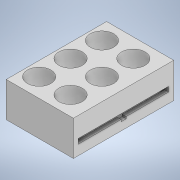
# Autodesk Inventor part: StirredVialHolder
Saved by Autodesk Inventor 2020 (Build 240168000, 168)
## iProperties
Created: 2021-07-14
Part Number: StirredVialHolder
Material: Generic
Document SubType Name: Modeling
Designer: pab2
Density: 1 g/cm^3
Appearance: Default
Author: pab2
Autodesk Inventor part; units mm, degrees
ref_plane "YZ Plane" through (0, 0, 0) normal (1, 0, 0) x (0, 1, 0)
ref_plane "XZ Plane" through (0, 0, 0) normal (0, 1, 0) x (-1, 0, 0)
ref_plane "XY Plane" through (0, 0, 0) normal (0, 0, 1) x (1, 0, 0)
sketch "Sketch1" plane through (0, 0, 0) normal (0, 1, 0) x (-1, 0, 0)
  line L0 (0, 0) -> (85.48, 0)
  line L1 (85.48, 0) -> (85.48, -127.76)
  line L2 (85.48, -127.76) -> (0, -127.76)
  line L3 (0, -127.76) -> (0, 0)
  line L4 (0, 0) -> (7.0711, -7.0711)
  line L5 (0, 0) -> (10, 0) construction
  circle A0 centre (7.0711, -7.0711) radius 4.7625
  dimension "d0" = 85.48
  dimension "d1" = 127.76
  dimension "offsetDiag" = 10
  dimension "d3" = 45
  dimension "d4" = 9.525
  constraints: 12 end point, 2 horizontal, 2 parallel, 1 centre point, 1 coincident, 1 equal length, 1 perpendicular
  measures "d0" distance of L1.end L2.end
  measures "d1" distance of L0.end L1.end
  measures "offsetDiag" distance of L0.start L4.end
  measures "d3" angle of L4 L5
  measures "d4" diameter of A0
extrude "Extrusion1" add sketch "Sketch1" along normal blind 12.7 contours L0 L1 L2 L3 | A0
sketch "Sketch3" plane through (0, 12.7, 0) normal (0, 1, 0) x (1, 0, 0)
  line L0 (0, 0) -> (0, 127.76) projected
  line L1 (0, 63.88) -> (-72.5, 63.88)
  line L2 (-140, 121.63) -> (-5, 121.63)
  line L3 (-5, 121.63) -> (-5, 6.13)
  line L4 (-5, 6.13) -> (-140, 6.13)
  line L5 (-140, 6.13) -> (-140, 121.63)
  line L6 (-140, 121.63) -> (-5, 6.13) construction
  line L7 (-5, 121.63) -> (-140, 6.13) construction
  dimension "d23" = 72.5
  dimension "d24" = 135
  dimension "d25" = 115.5
  constraints: 14 end point, 3 midpoint, 2 horizontal, 2 parallel, 1 perpendicular
  measures "d23" distance of L1.start L1.end
  measures "d24" distance of L3.end L4.end
  measures "d25" distance of L2.end L3.end
extrude "Extrusion2" cut sketch "Sketch3" against normal blind 2.54
sketch "Sketch4" plane through (0, 12.7, 0) normal (0, 1, 0) x (1, 0, 0)
  line L0 (-5, 121.63) -> (-5, 6.13) projected
  line L1 (5, 67.055) -> (-5, 67.055)
  line L2 (-5, 67.055) -> (-5, 60.705)
  line L3 (-5, 60.705) -> (5, 60.705)
  line L4 (5, 60.705) -> (5, 67.055)
  line L5 (0, 0) -> (0, 127.76) projected
  line L6 (5, 67.055) -> (-5, 60.705) construction
  line L7 (-5, 67.055) -> (5, 60.705) construction
  point P0 (0, 63.88)
  point P1 (0, 60.705)
  point P2 (0, 67.055)
  dimension "d28" = 6.35
  constraints: 12 end point, 3 midpoint, 2 parallel, 1 horizontal, 1 perpendicular, 1 point on line
  measures "d28" distance of L2.end L1.end
extrude "Extrusion3" cut sketch "Sketch4" against normal blind 2.54 contours L1 L5 L3 L0
sketch "Sketch5" plane through (0, 12.7, 0) normal (0, 1, 0) x (1, 0, 0)
  line L0 (0, 67.055) -> (0, 60.705) projected
  line L1 (0, 63.88) -> (-67.5, 63.88)
  circle A0 centre (-67.5, 63.88) radius 13.335
  line L2 (-85.48, 0) -> (0, 0) projected
  line L3 (-70.04, 127.76) -> (-38.29, 127.76)
  line L4 (-38.29, 127.76) -> (-38.29, 0)
  line L5 (-38.29, 0) -> (-70.04, 0)
  line L6 (-70.04, 0) -> (-70.04, 127.76)
  line L7 (-70.04, 127.76) -> (-38.29, 0) construction
  line L8 (-38.29, 127.76) -> (-70.04, 0) construction
  line L9 (-85.48, 121.63) -> (-5, 121.63) projected
  line L10 (-68.5166, 121.63) -> (-38.29, 121.63)
  line L11 (-38.29, 121.63) -> (-38.29, 127.76)
  line L12 (-38.29, 127.76) -> (-68.5166, 127.76)
  line L13 (-68.5166, 127.76) -> (-68.5166, 121.63)
  line L14 (-5, 6.13) -> (-85.48, 6.13) projected
  line L15 (-70.04, 0) -> (-38.29, 0)
  line L16 (-38.29, 0) -> (-38.29, 6.13)
  line L17 (-38.29, 6.13) -> (-70.04, 6.13)
  line L18 (-70.04, 6.13) -> (-70.04, 0)
  circle A1 centre (-67.5, 63.88) radius 14.9695
  point P0 (-54.165, 63.88)
  point P1 (-70.04, 6.13)
  point P2 (-38.29, 121.63)
  dimension "d32" = 26.67
  dimension "d31" = 67.5
  dimension "d33" = 31.75
  dimension "d158" = 29.939
  constraints: 30 end point, 6 parallel, 6 point on line, 4 horizontal, 3 midpoint, 3 perpendicular, 2 coincident, 1 centre point, 1 horizontal alignment, 2 other
  measures "d31" distance of L1.start L1.end
  measures "d33" distance of L4.end L5.end
  measures "d158" diameter of A1
sketch "Sketch22" plane through (0, 12.7, 0) normal (0, 1, 0) x (1, 0, 0)
  line L0 (0, 127.76) -> (-85.48, 127.76) projected
  line L1 (0, 0) -> (0, 127.76) projected
  line L2 (-85.48, 127.76) -> (0, 127.76)
  line L3 (0, 127.76) -> (0, 121.1763)
  line L4 (0, 121.1763) -> (-85.48, 121.1763)
  line L5 (-85.48, 121.1763) -> (-85.48, 127.76)
  line L6 (0, 0) -> (0, 60.705) projected
  line L7 (-5, 6.13) -> (-85.48, 6.13) projected
  line L8 (0, 0) -> (-85.48, 0)
  line L9 (-85.48, 0) -> (-85.48, 6.13)
  line L10 (-85.48, 6.13) -> (0, 6.13)
  line L11 (0, 6.13) -> (0, 0)
  constraints: 16 end point, 4 parallel, 2 horizontal, 2 perpendicular, 1 point on line
extrude "Extrusion16" add sketch "Sketch22" along normal blind 6.35
sketch "Sketch23" plane through (0, 19.05, 0) normal (0, 1, 0) x (1, 0, 0)
  line L0 (0, 127.76) -> (-85.48, 127.76) projected
  line L1 (-85.48, 0) -> (0, 0) projected
  line L2 (-85.48, 127.76) -> (0, 127.76)
  line L3 (0, 127.76) -> (0, 0)
  line L4 (0, 0) -> (-85.48, 0)
  line L5 (-85.48, 0) -> (-85.48, 127.76)
  constraints: 8 end point, 2 parallel, 1 horizontal, 1 perpendicular
extrude "Extrusion17" add sketch "Sketch23" along normal blind 25.4
extrude "Extrusion18" cut sketch "Sketch5" along normal blind 38.1 contours A1 L6 A0 L1 | L1 A0 L6 A1 | A0 L6 | L6 A0 A1 | L6 A0
pattern_linear "Rectangular Pattern2" count 3 spacing 40 along (0, 0, 1) count 2 spacing 40 along (1, 0, 0) of "Extrusion18" first direction both ways yes
sketch "Sketch24" plane through (-85.48, 0, -127.76) normal (-1, 0, 0) x (0, 0, 1)
  line L0 (121.63, 10.16) -> (6.13, 10.16) projected
  line L1 (63.88, 10.16) -> (63.88, 19.05)
  line L2 (78.8495, 19.05) -> (48.9105, 19.05) projected
  line L3 (6.13, 8.255) -> (121.63, 8.255)
  line L4 (121.63, 8.255) -> (121.63, 20.955)
  line L5 (121.63, 20.955) -> (6.13, 20.955)
  line L6 (6.13, 20.955) -> (6.13, 8.255)
  line L7 (6.13, 8.255) -> (121.63, 20.955) construction
  line L8 (121.63, 8.255) -> (6.13, 20.955) construction
  point P0 (127.76, 0)
  point P1 (63.88, 14.605)
  dimension "d167" = 12.7
  constraints: 14 end point, 5 midpoint, 2 parallel, 1 perpendicular
  measures "d167" distance of L4.end L3.end
extrude "Extrusion19" cut sketch "Sketch24" against normal up to surface (80.48 mm away)
body "Solid1"
